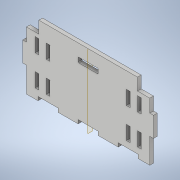
# Autodesk Inventor part: Side_one
Saved by Autodesk Inventor 2020 (Build 240168000, 168)
## iProperties
Created: 2019-12-17
Part Number: Side_one
Material: Generic
Document SubType Name: Modeling
Designer: fabfarm
Density: 1 g/cm^3
Appearance: Default
Author: fabfarm
Autodesk Inventor part; units mm, degrees
ref_plane "YZ Plane" through (0, 0, 0) normal (1, 0, 0) x (0, 1, 0)
ref_plane "XZ Plane" through (0, 0, 0) normal (0, 1, 0) x (-1, 0, 0)
ref_plane "XY Plane" through (0, 0, 0) normal (0, 0, 1) x (1, 0, 0)
sketch "Sketch1" plane through (0, 0, 0) normal (0, 0, 1) x (1, 0, 0)
  line L0 (0, 0) -> (-652, 0)
  line L1 (-652, 0) -> (-652, 350)
  line L2 (-652, 350) -> (0, 350)
  line L3 (0, 350) -> (0, 0)
  dimension "d0" = 350
  dimension "d1" = 652
  constraints: 8 end point, 2 parallel, 1 horizontal, 1 perpendicular
  measures "d0" distance of L2.end L0.start
  measures "d1" distance of L0.start L0.end
extrude "Extrusion1" add sketch "Sketch1" along normal blind 18.55
sketch "Sketch2" plane through (0, 0, 18.55) normal (0, 0, 1) x (1, 0, 0)
  line L0 (-652, 350) -> (-652, 0) projected
  line L1 (-652, 225) -> (-633.45, 225)
  line L2 (-633.45, 225) -> (-633.45, 350)
  line L3 (-633.45, 350) -> (-652, 350)
  line L4 (-652, 350) -> (-652, 225)
  line L5 (0, 350) -> (-652, 350) projected
  line L6 (-652, 0) -> (0, 0) projected
  line L7 (-652, 0) -> (-633.45, 0)
  line L8 (-633.45, 0) -> (-633.45, 125)
  line L9 (-633.45, 125) -> (-652, 125)
  line L10 (-652, 125) -> (-652, 0)
  dimension "d57" = 18.55
  dimension "d58" = 125
  dimension "d59" = 125
  constraints: 16 end point, 4 parallel, 2 collinear, 2 horizontal, 2 perpendicular, 1 point on line
  measures "d57" distance of L1.start L1.end
  measures "d58" distance of L3.end L1.start
  measures "d59" distance of L7.end L8.end
extrude "Extrusion2" cut sketch "Sketch2" against normal blind 18.55
ref_plane "Work Plane1" through (-326, 0, 0) normal (1, 0, 0) x (0, 0, -1)
mirror "Mirror1" about plane through (-326, 0, 0) normal (1, 0, 0) of "Extrusion2"
sketch "Sketch3" plane through (0, 0, 18.55) normal (0, 0, 1) x (1, 0, 0)
  line L0 (0, 350) -> (-652, 350) projected
  line L1 (-652, 290) -> (-572, 290)
  line L2 (-572, 290) -> (-572, 350)
  line L3 (-572, 350) -> (-652, 350)
  line L4 (-652, 350) -> (-652, 290)
  line L5 (-652, 330) -> (-652, 350) construction
  line L6 (-652, 350) -> (-633.45, 350) construction
  point P0 (0, 0)
  point P1 (-18.55, 350)
  dimension "d19" = 80
  dimension "d22" = 60
  constraints: 12 end point, 3 perpendicular, 1 parallel, 1 point on line, 1 vertical
  measures "d19" distance of L0.end L2.end
  measures "d22" distance of L0.end L1.start
extrude "Extrusion3" cut sketch "Sketch3" against normal blind 18.55
mirror "Mirror2" about plane through (-326, 0, 0) normal (1, 0, 0) of "Extrusion3"
sketch "Sketch4" plane through (0, 0, 18.55) normal (0, 0, 1) x (1, 0, 0)
  line L0 (-652, 0) -> (0, 0) projected
  line L1 (-652, 350) -> (-652, 0) projected
  line L2 (0, 0) -> (0, 350) projected
  line L3 (-576, 0) -> (-476, 0)
  line L4 (-476, 0) -> (-476, 18.55)
  line L5 (-476, 18.55) -> (-576, 18.55)
  line L6 (-576, 18.55) -> (-576, 0)
  line L7 (-376, 0) -> (-276, 0)
  line L8 (-276, 0) -> (-276, 18.55)
  line L9 (-276, 18.55) -> (-376, 18.55)
  line L10 (-376, 18.55) -> (-376, 0)
  line L11 (-176, 0) -> (-76, 0)
  line L12 (-76, 0) -> (-76, 18.55)
  line L13 (-76, 18.55) -> (-176, 18.55)
  line L14 (-176, 18.55) -> (-176, 0)
  dimension "d60" = 76
  dimension "d61" = 100
  dimension "d62" = 18.55
  dimension "d65" = 200
  dimension "d70" = 76
  constraints: 24 end point, 2 horizontal, 2 parallel, 1 perpendicular, 1 point on line, 16 other
  measures "d60" distance between parallel lines of L1 L6
  measures "d61" distance of L4.end L5.end
  measures "d62" distance of L3.end L4.end
  measures "d65" distance of L3.start L7.start
  measures "d70" distance between parallel lines of L2 L12
extrude "Extrusion4" cut sketch "Sketch4" against normal blind 20
sketch "Sketch5" plane through (0, 0, 18.55) normal (0, 0, 1) x (1, 0, 0)
  line L0 (-652, 30) -> (-633.45, 30)
  line L1 (-633.45, 30) -> (-633.45, 0)
  line L2 (-633.45, 0) -> (-652, 0)
  line L3 (-652, 0) -> (-652, 30)
  line L4 (-18.55, 30) -> (0, 30) projected
  line L5 (-18.55, 30) -> (0, 30)
  line L6 (0, 30) -> (0, 0)
  line L7 (0, 0) -> (-18.55, 0)
  line L8 (-18.55, 0) -> (-18.55, 30)
  line L9 (-633.45, 30) -> (-633.45, 10) projected
  line L10 (-652, 0) -> (-18.55, 0) projected
  point P0 (-611, 0)
  constraints: 16 end point, 4 parallel, 2 collinear, 2 horizontal, 2 perpendicular
extrude "Extrusion5" cut sketch "Sketch5" against normal blind 20
sketch "Sketch6" plane through (0, 0, 18.55) normal (0, 0, 1) x (1, 0, 0)
  line L0 (-276, 265) -> (-376, 265)
  line L1 (-376, 265) -> (-376, 290)
  line L2 (-376, 290) -> (-276, 290)
  line L3 (-276, 290) -> (-276, 265)
  line L4 (-276, 265) -> (-376, 290) construction
  line L5 (-376, 265) -> (-276, 290) construction
  line L6 (-326, 420) -> (-326, -70) projected
  line L7 (-80, 350) -> (-572, 350) projected
  point P0 (0, 0)
  point P1 (-326, 277.5)
  dimension "d38" = 25
  dimension "d39" = 100
  dimension "d40" = 60
  constraints: 12 end point, 2 midpoint, 2 parallel, 1 horizontal, 1 perpendicular, 1 point on line
  measures "d38" distance of L0.end L1.end
  measures "d39" distance of L1.end L2.end
  measures "d40" distance between parallel lines of L7 L2
extrude "Extrusion6" cut sketch "Sketch6" against normal blind 20
fillet "Fillet1" radius 4 4 edges at (-276, 290, 9.275) (-276, 265, 9.275) (-376, 290, 9.275) (-376, 265, 9.275)
sketch "Sketch7" plane through (0, 0, 18.55) normal (0, 0, 1) x (1, 0, 0)
  line L0 (-590.55, 48.55) -> (-572, 48.55)
  line L1 (-572, 48.55) -> (-572, 118.55)
  line L2 (-572, 118.55) -> (-590.55, 118.55)
  line L3 (-590.55, 118.55) -> (-590.55, 48.55)
  line L4 (-534.9, 48.55) -> (-516.35, 48.55)
  line L5 (-516.35, 48.55) -> (-516.35, 118.55)
  line L6 (-516.35, 118.55) -> (-534.9, 118.55)
  line L7 (-534.9, 118.55) -> (-534.9, 48.55)
  line L8 (-611, 18.55) -> (-591, 18.55) projected
  line L9 (-633.45, 70) -> (-633.45, 50) projected
  line L10 (-572, 350) -> (-572, 290) projected
  point P0 (0, 0)
  dimension "d44" = 37.1
  dimension "d45" = 18.55
  dimension "d46" = 70
  dimension "d47" = 30
  constraints: 16 end point, 4 parallel, 2 collinear, 2 horizontal, 2 perpendicular, 2 point on line
  measures "d44" distance between parallel lines of L7 L1
  measures "d45" distance of L1.end L2.end
  measures "d46" distance of L2.end L0.start
  measures "d47" distance between parallel lines of L8 L0
extrude "Extrusion7" cut sketch "Sketch7" against normal blind 20
mirror "Mirror3" about plane through (-326, 0, 0) normal (1, 0, 0) of "Extrusion7"
sketch "Esquisse8" plane through (0, 0, 0) normal (0, 0, -1) x (-1, 0, 0)
  line L0 (80, 200) -> (61.45, 200)
  line L1 (61.45, 200) -> (61.45, 270)
  line L2 (61.45, 270) -> (80, 270)
  line L3 (80, 270) -> (80, 200)
  line L4 (117.1, 270) -> (135.65, 270)
  line L5 (135.65, 270) -> (135.65, 200)
  line L6 (135.65, 200) -> (117.1, 200)
  line L7 (117.1, 200) -> (117.1, 270)
  line L8 (61.45, 48.55) -> (61.45, 118.55) projected
  line L9 (80, 118.55) -> (80, 48.55) projected
  line L10 (117.1, 48.55) -> (117.1, 118.55) projected
  line L11 (135.65, 118.55) -> (135.65, 48.55) projected
  line L12 (0, 270) -> (18.55, 270) projected
  point P0 (0, 0)
  dimension "d51" = 70
  constraints: 16 end point, 5 collinear, 4 parallel, 2 horizontal, 2 perpendicular, 2 point on line
  measures "d51" distance of L0.end L1.end
extrude "Extrusion8" cut sketch "Esquisse8" against normal blind 20
mirror "Symétrie4" about plane through (-326, 0, 0) normal (1, 0, 0) of "Extrusion8"
body "Solid1"
